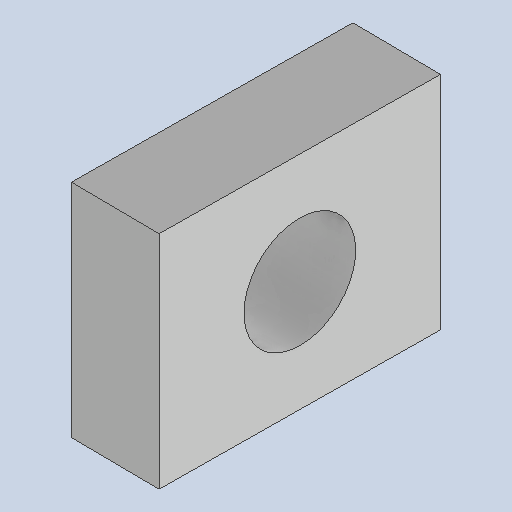
# Autodesk Inventor part: seilatrappeHalterMini
Saved by Autodesk Inventor 2025 (Build 290162010, 162A)
## iProperties
Created: 2024-11-20
Part Number: seilatrappeHalterMini
Material: Generisch
Document SubType Name: Modeling
Designer: Admin
Density: 1 g/cm^3
Appearance: Vorgabe
Author: Admin
Autodesk Inventor part; units mm, degrees
ref_plane "YZ Plane" through (0, 0, 0) normal (1, 0, 0) x (0, 1, 0)
ref_plane "XZ Plane" through (0, 0, 0) normal (0, 1, 0) x (-1, 0, 0)
ref_plane "XY Plane" through (0, 0, 0) normal (0, 0, 1) x (1, 0, 0)
sketch "Skizze1" plane through (0, 0, 0) normal (0, 0, 1) x (1, 0, 0)
  line L0 (-1.968335, -1.568021) -> (-1.93925, 1.431838)
  line L1 (-1.968335, -1.568021) -> (2.031477, -1.606801)
  line L2 (2.060562, 1.393058) -> (2.031477, -1.606801)
  line L3 (2.060562, 1.393058) -> (-1.93925, 1.431838)
  line L4 (-2.061408, -11.167569) -> (-2.032323, -8.16771)
  line L5 (-2.061408, -11.167569) -> (1.938404, -11.20635)
  line L6 (1.967489, -8.206491) -> (1.938404, -11.20635)
  line L7 (1.967489, -8.206491) -> (-2.032323, -8.16771)
  point P0 (0, 0)
extrude "Extrusion1" add sketch "Skizze1" along normal blind 10
sketch "Skizze2" plane through (-2.032323, -8.16771, 0) normal (0.0096951, 0.999953, 0) x (0.999953, -0.0096951, 0)
  line L0 (4, 0) -> (0, 0) projected
  line L1 (0, 0) -> (0, -10) projected
  line L2 (4, -10) -> (0, -10) projected
  line L3 (4, 0) -> (4, -10) projected
  point P0 (1.953041, 0)
extrude "Extrusion2" add sketch "Skizze2" along normal through all
sketch "Skizze3" plane through (-2.061408, -11.167569, 0) normal (-0.999953, 0.0096951, 0) x (0, 0, 1)
  arc A0 (5, 8.3) -> (5, 4.3) centre (5, 6.3) ccw
  point P0 (0, 11.18703)
  constraints: 2 point on circle, 1 centre point, 4 other
hole "Bohrung1" at (-2.000329, -4.867865, 5) direction (0.999953, -0.0096951, 0) diameter 5 end through all
